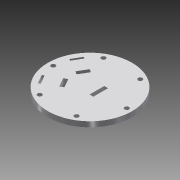
# Autodesk Inventor part: cap with wire cut
Saved by Autodesk Inventor 2015 (Build 190159000, 159)
## iProperties
Created: 2015-02-28
Part Number: cap with wire cut
Material: Generic
Document SubType Name: Modeling
Designer: Qiuyang
Density: 1 g/cm^3
Appearance: Default
Author: Qiuyang
Autodesk Inventor part; units mm, degrees
ref_plane "YZ Plane" through (0, 0, 0) normal (1, 0, 0) x (0, 1, 0)
ref_plane "XZ Plane" through (0, 0, 0) normal (0, 1, 0) x (-1, 0, 0)
ref_plane "XY Plane" through (0, 0, 0) normal (0, 0, 1) x (1, 0, 0)
sketch "Sketch4" plane through (0, 0, 0) normal (0, 1, 0) x (-1, 0, 0)
  circle A0 centre (0, 0) radius 50.8
  dimension "d2" = 101.6
  constraints: 1 centre point, 1 coincident
  measures "d2" diameter of A0
extrude "Extrusion3" add sketch "Sketch4" along normal blind 6.35
sketch "Sketch10" plane through (0, 6.35, 0) normal (0, 1, 0) x (1, 0, 0)
  circle A0 centre (-44.462, 0) radius 2.667
  circle A1 centre (-22.231, -38.5052) radius 2.667
  circle A2 centre (22.231, -38.5052) radius 2.667
  circle A3 centre (44.462, 0) radius 2.667
  circle A4 centre (22.231, 38.5052) radius 2.667
  circle A5 centre (-22.231, 38.5052) radius 2.667
  point P0 (0, 0)
  dimension "d48" = 5.334
  dimension "d51" = 360
  constraints: 6 centre point, 13 other
  measures "d48" diameter of A0
extrude "Extrusion6" cut sketch "Sketch10" against normal blind 6.35
sketch "Sketch13" plane through (0, 6.35, 0) normal (0, 1, 0) x (1, 0, 0)
  line L0 (-25.3494, -7.0256) -> (-21.3685, -4.7771)
  line L1 (-21.3685, -4.7771) -> (-15.1225, -15.8349)
  line L2 (-15.1225, -15.8349) -> (-19.1033, -18.0835)
  line L3 (-19.1033, -18.0835) -> (-25.3494, -7.0256)
  line L4 (-25.3494, -7.0256) -> (-21.3685, -4.7771)
  line L5 (-21.3685, -4.7771) -> (-15.1225, -15.8349)
  line L6 (-15.1225, -15.8349) -> (-19.1033, -18.0835)
  line L7 (-19.1033, -18.0835) -> (-25.3494, -7.0256)
  line L8 (-25.3494, -7.0256) -> (-21.3685, -4.7771)
  line L9 (-21.3685, -4.7771) -> (-15.1225, -15.8349)
  line L10 (-15.1225, -15.8349) -> (-19.1033, -18.0835)
  line L11 (-19.1033, -18.0835) -> (-25.3494, -7.0256)
  line L12 (-25.3494, -7.0256) -> (-21.3685, -4.7771)
  line L13 (-21.3685, -4.7771) -> (-15.1225, -15.8349)
  line L14 (-15.1225, -15.8349) -> (-19.1033, -18.0835)
  line L15 (-19.1033, -18.0835) -> (-25.3494, -7.0256)
  line L16 (-25.3494, -7.0256) -> (-21.3685, -4.7771)
  line L17 (-21.3685, -4.7771) -> (-15.1225, -15.8349)
  line L18 (-15.1225, -15.8349) -> (-19.1033, -18.0835)
  line L19 (-19.1033, -18.0835) -> (-25.3494, -7.0256)
  line L20 (-25.3494, -7.0256) -> (-21.3685, -4.7771)
  line L21 (-21.3685, -4.7771) -> (-15.1225, -15.8349)
  line L22 (-15.1225, -15.8349) -> (-19.1033, -18.0835)
  line L23 (-19.1033, -18.0835) -> (-25.3494, -7.0256)
  line L24 (-18.7591, 18.4404) -> (-14.8213, 16.1172)
  line L25 (-14.8213, 16.1172) -> (-21.2747, 5.179)
  line L26 (-21.2747, 5.179) -> (-25.2124, 7.5022)
  line L27 (-25.2124, 7.5022) -> (-18.7591, 18.4404)
  line L28 (-18.7591, 18.4404) -> (-14.8213, 16.1172)
  line L29 (-14.8213, 16.1172) -> (-21.2747, 5.179)
  line L30 (-21.2747, 5.179) -> (-25.2124, 7.5022)
  line L31 (-25.2124, 7.5022) -> (-18.7591, 18.4404)
  line L32 (-18.7591, 18.4404) -> (-14.8213, 16.1172)
  line L33 (-14.8213, 16.1172) -> (-21.2747, 5.179)
  line L34 (-21.2747, 5.179) -> (-25.2124, 7.5022)
  line L35 (-25.2124, 7.5022) -> (-18.7591, 18.4404)
  line L36 (-18.7591, 18.4404) -> (-14.8213, 16.1172)
  line L37 (-14.8213, 16.1172) -> (-21.2747, 5.179)
  line L38 (-21.2747, 5.179) -> (-25.2124, 7.5022)
  line L39 (-25.2124, 7.5022) -> (-18.7591, 18.4404)
  line L40 (-18.7591, 18.4404) -> (-14.8213, 16.1172)
  line L41 (-14.8213, 16.1172) -> (-21.2747, 5.179)
  line L42 (-21.2747, 5.179) -> (-25.2124, 7.5022)
  line L43 (-25.2124, 7.5022) -> (-18.7591, 18.4404)
  line L44 (-18.7591, 18.4404) -> (-14.8213, 16.1172)
  line L45 (-14.8213, 16.1172) -> (-21.2747, 5.179)
  line L46 (-21.2747, 5.179) -> (-25.2124, 7.5022)
  line L47 (-25.2124, 7.5022) -> (-18.7591, 18.4404)
  line L48 (7.62, 9.652) -> (12.192, 9.652)
  line L49 (12.192, 9.652) -> (12.192, -8.128)
  line L50 (12.192, -8.128) -> (7.62, -8.128)
  line L51 (7.62, -8.128) -> (7.62, 9.652)
  line L52 (-41.7125, -16.7155) -> (-39.5128, -15.4455)
  line L53 (-39.5128, -15.4455) -> (-33.1628, -26.444)
  line L54 (-33.1628, -26.444) -> (-35.3625, -27.714)
  line L55 (-35.3625, -27.714) -> (-41.7125, -16.7155)
  line L56 (-35.3322, 27.7663) -> (-33.1325, 26.4963)
  line L57 (-33.1325, 26.4963) -> (-39.4825, 15.4978)
  line L58 (-39.4825, 15.4978) -> (-41.6822, 16.7678)
  line L59 (-41.6822, 16.7678) -> (-35.3322, 27.7663)
  point P0 (0, 0)
  dimension "d57" = 4.572
  dimension "d58" = 12.7
  dimension "d59" = 4.572
  dimension "d60" = 12.7
  dimension "d61" = 4.572
  dimension "d62" = 12.7
  dimension "d63" = 4.572
  dimension "d64" = 12.7
  dimension "d65" = 4.572
  dimension "d66" = 12.7
  dimension "d67" = 4.572
  dimension "d68" = 12.7
  dimension "d69" = 4.572
  dimension "d70" = 12.7
  dimension "d71" = 4.572
  dimension "d72" = 12.7
  dimension "d73" = 4.572
  dimension "d74" = 12.7
  dimension "d75" = 4.572
  dimension "d76" = 12.7
  dimension "d77" = 4.572
  dimension "d78" = 12.7
  dimension "d79" = 4.572
  dimension "d80" = 12.7
  dimension "d81" = 4.572
  dimension "d82" = 17.78
  dimension "d109" = 2.54
  dimension "d110" = 12.7
  dimension "d113" = 2.54
  dimension "d114" = 12.7
  constraints: 120 end point, 30 parallel, 15 perpendicular, 1 horizontal
  measures "d57" distance of L1.end L2.end
  measures "d58" distance of L0.end L1.end
  measures "d59" distance of L5.end L6.end
  measures "d60" distance of L4.end L5.end
  measures "d61" distance of L9.end L10.end
  measures "d62" distance of L8.end L9.end
  measures "d63" distance of L13.end L14.end
  measures "d64" distance of L12.end L13.end
  measures "d65" distance of L17.end L18.end
  measures "d66" distance of L16.end L17.end
  measures "d67" distance of L21.end L22.end
  measures "d68" distance of L20.end L21.end
  measures "d69" distance of L25.end L27.start
  measures "d70" distance of L25.start L25.end
  measures "d71" distance of L29.end L31.start
  measures "d72" distance of L29.start L29.end
  measures "d73" distance of L33.end L35.start
  measures "d74" distance of L33.start L33.end
  measures "d75" distance of L37.end L39.start
  measures "d76" distance of L37.start L37.end
  measures "d77" distance of L41.end L43.start
  measures "d78" distance of L41.start L41.end
  measures "d79" distance of L45.end L47.start
  measures "d80" distance of L45.start L45.end
  measures "d81" distance of L49.end L50.end
  measures "d82" distance of L48.end L49.end
  measures "d109" distance of L53.end L54.end
  measures "d110" distance of L52.end L53.end
  measures "d113" distance of L58.start L58.end
  measures "d114" distance of L56.end L58.start
extrude "Extrusion8" cut sketch "Sketch13" against normal blind 6.35
body "Solid3"
